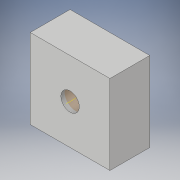
# Autodesk Inventor part: socket
Saved by Autodesk Inventor 2019 (Build 230136000, 136)
## iProperties
Created: 2018-07-14
Part Number: socket
Material: Generic
Document SubType Name: Modeling
Designer: steele
Density: 1 g/cm^3
Appearance: Default
Author: steele
Autodesk Inventor part; units mm, degrees
ref_plane "YZ Plane" through (0, 0, 0) normal (1, 0, 0) x (0, 1, 0)
ref_plane "XZ Plane" through (0, 0, 0) normal (0, 1, 0) x (-1, 0, 0)
ref_plane "XY Plane" through (0, 0, 0) normal (0, 0, 1) x (1, 0, 0)
sketch "Sketch1" plane through (0, 0, 0) normal (0, 0, 1) x (1, 0, 0)
  line L0 (-25.4, -25.4) -> (25.4, -25.4)
  line L1 (25.4, -25.4) -> (25.4, 25.4)
  line L2 (25.4, 25.4) -> (-25.4, 25.4)
  line L3 (-25.4, 25.4) -> (-25.4, -25.4)
  line L4 (-25.4, -25.4) -> (25.4, 25.4) construction
  line L5 (25.4, -25.4) -> (-25.4, 25.4) construction
  point P0 (0, 0)
  dimension "d0" = 50.8
  constraints: 12 end point, 2 midpoint, 2 parallel, 2 perpendicular, 1 horizontal
  measures "d0" distance of L0.end L1.end
extrude "Extrusion1" add sketch "Sketch1" along normal mid plane 25.4
ref_plane "Work Plane1" through (0, 0, 9.525) normal (0, 0, 1) x (1, 0, 0)
sketch "Sketch2" plane through (0, 0, 9.525) normal (0, 0, 1) x (1, 0, 0)
  arc A0 (0, -6.6675) -> (0, 6.6675) centre (0, 0) ccw
  line L0 (0, -6.6675) -> (0, 6.6675)
  dimension "d5" = 6.6675
  constraints: 2 end point, 2 point on circle, 1 centre point, 1 coincident
  measures "d5" radius of A0
revolve "Revolution1" cut sketch "Sketch2" angle 360 about axis through (0, -6.6675, 9.525) along (0, 1, 0)
equation "\"d0\" = sideLength"
equation "\"d1\" = partDepth"
equation "\"d5\" = radiusofBallHole"
equation "\"d3\" = -workPlaneForBallDistanceFfromFontEdge"
equation "\"radiusofBallHole\" = 0.5 * diameterOfBallHole"
equation "\"sideLength\" = 50.8"
equation "\"partDepth\" = 25.4"
equation "\"workPlaneForBallDistanceFfromFontEdge\" = 3.175"
equation "\"allowancForBallToRotate\" = 0.635"
equation "\"diameterOfBallHole\" = 13.335"
body "Solid1"
